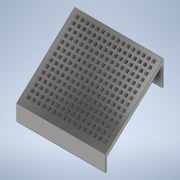
# Autodesk Inventor part: Rejilla_4x4mm
Saved by Autodesk Inventor 2021 (Build 250183000, 183)
## iProperties
Created: 2021-06-27
Part Number: Rejilla_4x4mm
Material: Acero inoxidable
Document SubType Name: Modeling
Designer: artur
Density: 8 g/cm^3
Appearance: Acero - Pulido
Mass: 658.868 g
Surface Area: 625.183 cm^2
Volume: 82.3585 cm^3
Author: artur
Autodesk Inventor part; units mm, degrees
ref_plane "YZ Plane" through (0, 0, 0) normal (1, 0, 0) x (0, 1, 0)
ref_plane "XZ Plane" through (0, 0, 0) normal (0, 1, 0) x (-1, 0, 0)
ref_plane "XY Plane" through (0, 0, 0) normal (0, 0, 1) x (1, 0, 0)
sketch "Boceto6" plane through (-46.053, -27.9809, 0) normal (0, 0, 1) x (1, 0, 0)
  line L0 (118.929, 0) -> (171.1141, 0) construction
  line L1 (-1.0005, -0.9307) -> (-79.0081, -0.9307) construction
  line L2 (-1.0005, -0.9307) -> (89.9995, 83.721)
  line L3 (-1.0005, -0.9307) -> (-1.0005, -25.8991)
  line L4 (-1.0005, -25.8991) -> (0.9995, -25.8991)
  line L5 (0.9995, -25.8991) -> (0.9995, -5.8991)
  line L6 (80.5422, 57.5078) -> (86.2007, 57.5078)
  line L7 (89.9995, 83.721) -> (89.9995, 45.0316)
  line L8 (89.9995, 45.0316) -> (87.9995, 45.0316)
  line L9 (87.9995, 45.0316) -> (87.9995, 75.0316)
  line L10 (0.9995, -5.8991) -> (87.9995, 75.0316)
  dimension "d69" = 137.07
  dimension "d66" = 2
  dimension "d65" = 5
  dimension "d64" = 30
  dimension "d62" = 2
  dimension "d68" = 5
  dimension "d67" = 20
  dimension "d93" = 89
  constraints: 22 end point, 4 horizontal, 2 perpendicular, 2 vertical
  measures "d69" angle of L1 L2
  measures "d66" distance between parallel lines of L5 L3
  measures "d65" distance from line of L2 L9.end
  measures "d64" distance of L8.end L9.end
  measures "d62" distance between parallel lines of L7 L9
  measures "d68" distance from line of L2 L5.end
  measures "d67" distance of L4.end L5.end
  measures "d93" distance between parallel lines of L3 L9
extrude "Extrusión5" add sketch "Boceto6" along normal blind 139
sketch "Boceto7" plane through (-47.0535, -28.9116, 139) normal (-0.6811, 0.7322, 0) x (0.7322, 0.6811, 0)
  line L0 (118.2856, 131) -> (114.2856, 131)
  line L1 (114.2856, 131) -> (114.2856, 127)
  line L2 (114.2856, 127) -> (118.2856, 127)
  line L3 (118.2856, 127) -> (118.2856, 131)
  line L4 (124.2856, 139) -> (124.2856, 0) projected
  line L5 (124.2856, 139) -> (0, 139) projected
  line L6 (118.2856, 123) -> (114.2856, 123)
  line L7 (114.2856, 123) -> (114.2856, 119)
  line L8 (114.2856, 119) -> (118.2856, 119)
  line L9 (118.2856, 119) -> (118.2856, 123)
  line L10 (118.2856, 115) -> (114.2856, 115)
  line L11 (114.2856, 115) -> (114.2856, 111)
  line L12 (114.2856, 111) -> (118.2856, 111)
  line L13 (118.2856, 111) -> (118.2856, 115)
  line L14 (118.2856, 107) -> (114.2856, 107)
  line L15 (114.2856, 107) -> (114.2856, 103)
  line L16 (114.2856, 103) -> (118.2856, 103)
  line L17 (118.2856, 103) -> (118.2856, 107)
  line L18 (118.2856, 99) -> (114.2856, 99)
  line L19 (114.2856, 99) -> (114.2856, 95)
  line L20 (114.2856, 95) -> (118.2856, 95)
  line L21 (118.2856, 95) -> (118.2856, 99)
  line L22 (118.2856, 91) -> (114.2856, 91)
  line L23 (114.2856, 91) -> (114.2856, 87)
  line L24 (114.2856, 87) -> (118.2856, 87)
  line L25 (118.2856, 87) -> (118.2856, 91)
  line L26 (118.2856, 83) -> (114.2856, 83)
  line L27 (114.2856, 83) -> (114.2856, 79)
  line L28 (114.2856, 79) -> (118.2856, 79)
  line L29 (118.2856, 79) -> (118.2856, 83)
  line L30 (118.2856, 75) -> (114.2856, 75)
  line L31 (114.2856, 75) -> (114.2856, 71)
  line L32 (114.2856, 71) -> (118.2856, 71)
  line L33 (118.2856, 71) -> (118.2856, 75)
  line L34 (118.2856, 67) -> (114.2856, 67)
  line L35 (114.2856, 67) -> (114.2856, 63)
  line L36 (114.2856, 63) -> (118.2856, 63)
  line L37 (118.2856, 63) -> (118.2856, 67)
  line L38 (118.2856, 59) -> (114.2856, 59)
  line L39 (114.2856, 59) -> (114.2856, 55)
  line L40 (114.2856, 55) -> (118.2856, 55)
  line L41 (118.2856, 55) -> (118.2856, 59)
  line L42 (118.2856, 51) -> (114.2856, 51)
  line L43 (114.2856, 51) -> (114.2856, 47)
  line L44 (114.2856, 47) -> (118.2856, 47)
  line L45 (118.2856, 47) -> (118.2856, 51)
  line L46 (118.2856, 43) -> (114.2856, 43)
  line L47 (114.2856, 43) -> (114.2856, 39)
  line L48 (114.2856, 39) -> (118.2856, 39)
  line L49 (118.2856, 39) -> (118.2856, 43)
  line L50 (118.2856, 35) -> (114.2856, 35)
  line L51 (114.2856, 35) -> (114.2856, 31)
  line L52 (114.2856, 31) -> (118.2856, 31)
  line L53 (118.2856, 31) -> (118.2856, 35)
  line L54 (118.2856, 27) -> (114.2856, 27)
  line L55 (114.2856, 27) -> (114.2856, 23)
  line L56 (114.2856, 23) -> (118.2856, 23)
  line L57 (118.2856, 23) -> (118.2856, 27)
  line L58 (118.2856, 19) -> (114.2856, 19)
  line L59 (114.2856, 19) -> (114.2856, 15)
  line L60 (114.2856, 15) -> (118.2856, 15)
  line L61 (118.2856, 15) -> (118.2856, 19)
  line L62 (118.2856, 11) -> (114.2856, 11)
  line L63 (114.2856, 11) -> (114.2856, 7)
  line L64 (114.2856, 7) -> (118.2856, 7)
  line L65 (118.2856, 7) -> (118.2856, 11)
  line L66 (110.2856, 127) -> (110.2856, 131)
  line L67 (110.2856, 131) -> (106.2856, 131)
  line L68 (106.2856, 131) -> (106.2856, 127)
  line L69 (106.2856, 123) -> (106.2856, 119)
  line L70 (106.2856, 119) -> (110.2856, 119)
  line L71 (110.2856, 119) -> (110.2856, 123)
  line L72 (110.2856, 115) -> (106.2856, 115)
  line L73 (110.2856, 111) -> (110.2856, 115)
  line L74 (106.2856, 115) -> (106.2856, 111)
  line L75 (106.2856, 111) -> (110.2856, 111)
  line L76 (110.2856, 107) -> (106.2856, 107)
  line L77 (106.2856, 103) -> (110.2856, 103)
  line L78 (106.2856, 107) -> (106.2856, 103)
  line L79 (110.2856, 103) -> (110.2856, 107)
  line L80 (106.2856, 127) -> (110.2856, 127)
  line L81 (110.2856, 123) -> (106.2856, 123)
  line L82 (110.2856, 99) -> (106.2856, 99)
  line L83 (106.2856, 99) -> (106.2856, 95)
  line L84 (110.2856, 95) -> (110.2856, 99)
  line L85 (110.2856, 91) -> (106.2856, 91)
  line L86 (106.2856, 87) -> (110.2856, 87)
  line L87 (110.2856, 87) -> (110.2856, 91)
  line L88 (106.2856, 91) -> (106.2856, 87)
  line L89 (106.2856, 95) -> (110.2856, 95)
  line L90 (110.2856, 83) -> (106.2856, 83)
  line L91 (106.2856, 83) -> (106.2856, 79)
  line L92 (110.2856, 79) -> (110.2856, 83)
  line L93 (106.2856, 79) -> (110.2856, 79)
  line L94 (110.2856, 75) -> (106.2856, 75)
  line L95 (106.2856, 75) -> (106.2856, 71)
  line L96 (110.2856, 71) -> (110.2856, 75)
  line L97 (106.2856, 71) -> (110.2856, 71)
  line L98 (106.2856, 63) -> (110.2856, 63)
  line L99 (110.2856, 63) -> (110.2856, 67)
  line L100 (106.2856, 67) -> (106.2856, 63)
  line L101 (110.2856, 67) -> (106.2856, 67)
  line L102 (110.2856, 59) -> (106.2856, 59)
  line L103 (106.2856, 59) -> (106.2856, 55)
  line L104 (110.2856, 55) -> (110.2856, 59)
  line L105 (106.2856, 55) -> (110.2856, 55)
  line L106 (110.2856, 51) -> (106.2856, 51)
  line L107 (106.2856, 51) -> (106.2856, 47)
  line L108 (106.2856, 47) -> (110.2856, 47)
  line L109 (110.2856, 47) -> (110.2856, 51)
  line L110 (110.2856, 43) -> (106.2856, 43)
  line L111 (106.2856, 43) -> (106.2856, 39)
  line L112 (110.2856, 39) -> (110.2856, 43)
  line L113 (106.2856, 39) -> (110.2856, 39)
  line L114 (110.2856, 35) -> (106.2856, 35)
  line L115 (110.2856, 31) -> (110.2856, 35)
  line L116 (106.2856, 31) -> (110.2856, 31)
  line L117 (106.2856, 35) -> (106.2856, 31)
  line L118 (110.2856, 27) -> (106.2856, 27)
  line L119 (106.2856, 27) -> (106.2856, 23)
  line L120 (110.2856, 23) -> (110.2856, 27)
  line L121 (106.2856, 23) -> (110.2856, 23)
  line L122 (110.2856, 19) -> (106.2856, 19)
  line L123 (106.2856, 19) -> (106.2856, 15)
  line L124 (106.2856, 15) -> (110.2856, 15)
  line L125 (110.2856, 15) -> (110.2856, 19)
  line L126 (110.2856, 11) -> (106.2856, 11)
  line L127 (106.2856, 11) -> (106.2856, 7)
  line L128 (106.2856, 7) -> (110.2856, 7)
  line L129 (110.2856, 7) -> (110.2856, 11)
  line L130 (102.2856, 127) -> (102.2856, 131)
  line L131 (102.2856, 131) -> (98.2856, 131)
  line L132 (98.2856, 131) -> (98.2856, 127)
  line L133 (98.2856, 123) -> (98.2856, 119)
  line L134 (98.2856, 119) -> (102.2856, 119)
  line L135 (102.2856, 119) -> (102.2856, 123)
  line L136 (102.2856, 115) -> (98.2856, 115)
  line L137 (102.2856, 111) -> (102.2856, 115)
  line L138 (98.2856, 115) -> (98.2856, 111)
  line L139 (98.2856, 111) -> (102.2856, 111)
  line L140 (102.2856, 107) -> (98.2856, 107)
  line L141 (98.2856, 103) -> (102.2856, 103)
  line L142 (98.2856, 107) -> (98.2856, 103)
  line L143 (102.2856, 103) -> (102.2856, 107)
  line L144 (98.2856, 127) -> (102.2856, 127)
  line L145 (102.2856, 123) -> (98.2856, 123)
  line L146 (102.2856, 99) -> (98.2856, 99)
  line L147 (98.2856, 99) -> (98.2856, 95)
  line L148 (102.2856, 95) -> (102.2856, 99)
  line L149 (102.2856, 91) -> (98.2856, 91)
  line L150 (98.2856, 87) -> (102.2856, 87)
  line L151 (102.2856, 87) -> (102.2856, 91)
  line L152 (98.2856, 91) -> (98.2856, 87)
  line L153 (98.2856, 95) -> (102.2856, 95)
  line L154 (102.2856, 83) -> (98.2856, 83)
  line L155 (98.2856, 83) -> (98.2856, 79)
  line L156 (102.2856, 79) -> (102.2856, 83)
  line L157 (98.2856, 79) -> (102.2856, 79)
  line L158 (102.2856, 75) -> (98.2856, 75)
  line L159 (98.2856, 75) -> (98.2856, 71)
  line L160 (102.2856, 71) -> (102.2856, 75)
  line L161 (98.2856, 71) -> (102.2856, 71)
  line L162 (98.2856, 63) -> (102.2856, 63)
  line L163 (102.2856, 63) -> (102.2856, 67)
  line L164 (98.2856, 67) -> (98.2856, 63)
  line L165 (102.2856, 67) -> (98.2856, 67)
  line L166 (102.2856, 59) -> (98.2856, 59)
  line L167 (98.2856, 59) -> (98.2856, 55)
  line L168 (102.2856, 55) -> (102.2856, 59)
  line L169 (98.2856, 55) -> (102.2856, 55)
  line L170 (102.2856, 51) -> (98.2856, 51)
  line L171 (98.2856, 51) -> (98.2856, 47)
  line L172 (98.2856, 47) -> (102.2856, 47)
  line L173 (102.2856, 47) -> (102.2856, 51)
  line L174 (102.2856, 43) -> (98.2856, 43)
  line L175 (98.2856, 43) -> (98.2856, 39)
  line L176 (102.2856, 39) -> (102.2856, 43)
  line L177 (98.2856, 39) -> (102.2856, 39)
  line L178 (102.2856, 35) -> (98.2856, 35)
  line L179 (102.2856, 31) -> (102.2856, 35)
  line L180 (98.2856, 31) -> (102.2856, 31)
  line L181 (98.2856, 35) -> (98.2856, 31)
  line L182 (102.2856, 27) -> (98.2856, 27)
  line L183 (98.2856, 27) -> (98.2856, 23)
  line L184 (102.2856, 23) -> (102.2856, 27)
  line L185 (98.2856, 23) -> (102.2856, 23)
  line L186 (102.2856, 19) -> (98.2856, 19)
  line L187 (98.2856, 19) -> (98.2856, 15)
  line L188 (98.2856, 15) -> (102.2856, 15)
  line L189 (102.2856, 15) -> (102.2856, 19)
  line L190 (102.2856, 11) -> (98.2856, 11)
  line L191 (98.2856, 11) -> (98.2856, 7)
  line L192 (98.2856, 7) -> (102.2856, 7)
  line L193 (102.2856, 7) -> (102.2856, 11)
  line L194 (94.2856, 127) -> (94.2856, 131)
  line L195 (94.2856, 131) -> (90.2856, 131)
  line L196 (90.2856, 131) -> (90.2856, 127)
  line L197 (90.2856, 123) -> (90.2856, 119)
  line L198 (90.2856, 119) -> (94.2856, 119)
  line L199 (94.2856, 119) -> (94.2856, 123)
  line L200 (94.2856, 115) -> (90.2856, 115)
  line L201 (94.2856, 111) -> (94.2856, 115)
  line L202 (90.2856, 115) -> (90.2856, 111)
  line L203 (90.2856, 111) -> (94.2856, 111)
  line L204 (94.2856, 107) -> (90.2856, 107)
  line L205 (90.2856, 103) -> (94.2856, 103)
  line L206 (90.2856, 107) -> (90.2856, 103)
  line L207 (94.2856, 103) -> (94.2856, 107)
  line L208 (90.2856, 127) -> (94.2856, 127)
  line L209 (94.2856, 123) -> (90.2856, 123)
  line L210 (94.2856, 99) -> (90.2856, 99)
  line L211 (90.2856, 99) -> (90.2856, 95)
  line L212 (94.2856, 95) -> (94.2856, 99)
  line L213 (94.2856, 91) -> (90.2856, 91)
  line L214 (90.2856, 87) -> (94.2856, 87)
  line L215 (94.2856, 87) -> (94.2856, 91)
  line L216 (90.2856, 91) -> (90.2856, 87)
  line L217 (90.2856, 95) -> (94.2856, 95)
  line L218 (94.2856, 83) -> (90.2856, 83)
  line L219 (90.2856, 83) -> (90.2856, 79)
  line L220 (94.2856, 79) -> (94.2856, 83)
  line L221 (90.2856, 79) -> (94.2856, 79)
  line L222 (94.2856, 75) -> (90.2856, 75)
  line L223 (90.2856, 75) -> (90.2856, 71)
  line L224 (94.2856, 71) -> (94.2856, 75)
  line L225 (90.2856, 71) -> (94.2856, 71)
  line L226 (90.2856, 63) -> (94.2856, 63)
  line L227 (94.2856, 63) -> (94.2856, 67)
  line L228 (90.2856, 67) -> (90.2856, 63)
  line L229 (94.2856, 67) -> (90.2856, 67)
  line L230 (94.2856, 59) -> (90.2856, 59)
  line L231 (90.2856, 59) -> (90.2856, 55)
  line L232 (94.2856, 55) -> (94.2856, 59)
  line L233 (90.2856, 55) -> (94.2856, 55)
  line L234 (94.2856, 51) -> (90.2856, 51)
  line L235 (90.2856, 51) -> (90.2856, 47)
  line L236 (90.2856, 47) -> (94.2856, 47)
  line L237 (94.2856, 47) -> (94.2856, 51)
  line L238 (94.2856, 43) -> (90.2856, 43)
  line L239 (90.2856, 43) -> (90.2856, 39)
  line L240 (94.2856, 39) -> (94.2856, 43)
  line L241 (90.2856, 39) -> (94.2856, 39)
  line L242 (94.2856, 35) -> (90.2856, 35)
  line L243 (94.2856, 31) -> (94.2856, 35)
  line L244 (90.2856, 31) -> (94.2856, 31)
  line L245 (90.2856, 35) -> (90.2856, 31)
  line L246 (94.2856, 27) -> (90.2856, 27)
  line L247 (90.2856, 27) -> (90.2856, 23)
  line L248 (94.2856, 23) -> (94.2856, 27)
  line L249 (90.2856, 23) -> (94.2856, 23)
  line L250 (94.2856, 19) -> (90.2856, 19)
  line L251 (90.2856, 19) -> (90.2856, 15)
  line L252 (90.2856, 15) -> (94.2856, 15)
  line L253 (94.2856, 15) -> (94.2856, 19)
  line L254 (94.2856, 11) -> (90.2856, 11)
  line L255 (90.2856, 11) -> (90.2856, 7)
  line L256 (90.2856, 7) -> (94.2856, 7)
  line L257 (94.2856, 7) -> (94.2856, 11)
  line L258 (86.2856, 127) -> (86.2856, 131)
  line L259 (86.2856, 131) -> (82.2856, 131)
  line L260 (82.2856, 131) -> (82.2856, 127)
  line L261 (82.2856, 123) -> (82.2856, 119)
  line L262 (82.2856, 119) -> (86.2856, 119)
  line L263 (86.2856, 119) -> (86.2856, 123)
  line L264 (86.2856, 115) -> (82.2856, 115)
  line L265 (86.2856, 111) -> (86.2856, 115)
  line L266 (82.2856, 115) -> (82.2856, 111)
  line L267 (82.2856, 111) -> (86.2856, 111)
  line L268 (86.2856, 107) -> (82.2856, 107)
  line L269 (82.2856, 103) -> (86.2856, 103)
  line L270 (82.2856, 107) -> (82.2856, 103)
  line L271 (86.2856, 103) -> (86.2856, 107)
  line L272 (82.2856, 127) -> (86.2856, 127)
  line L273 (86.2856, 123) -> (82.2856, 123)
  line L274 (86.2856, 99) -> (82.2856, 99)
  line L275 (82.2856, 99) -> (82.2856, 95)
  line L276 (86.2856, 95) -> (86.2856, 99)
  line L277 (86.2856, 91) -> (82.2856, 91)
  line L278 (82.2856, 87) -> (86.2856, 87)
  line L279 (86.2856, 87) -> (86.2856, 91)
  line L280 (82.2856, 91) -> (82.2856, 87)
  line L281 (82.2856, 95) -> (86.2856, 95)
  line L282 (86.2856, 83) -> (82.2856, 83)
  line L283 (82.2856, 83) -> (82.2856, 79)
  line L284 (86.2856, 79) -> (86.2856, 83)
  line L285 (82.2856, 79) -> (86.2856, 79)
  line L286 (86.2856, 75) -> (82.2856, 75)
  line L287 (82.2856, 75) -> (82.2856, 71)
  line L288 (86.2856, 71) -> (86.2856, 75)
  line L289 (82.2856, 71) -> (86.2856, 71)
  line L290 (82.2856, 63) -> (86.2856, 63)
  line L291 (86.2856, 63) -> (86.2856, 67)
  line L292 (82.2856, 67) -> (82.2856, 63)
  line L293 (86.2856, 67) -> (82.2856, 67)
  line L294 (86.2856, 59) -> (82.2856, 59)
  line L295 (82.2856, 59) -> (82.2856, 55)
  line L296 (86.2856, 55) -> (86.2856, 59)
  line L297 (82.2856, 55) -> (86.2856, 55)
  line L298 (86.2856, 51) -> (82.2856, 51)
  line L299 (82.2856, 51) -> (82.2856, 47)
  line L300 (82.2856, 47) -> (86.2856, 47)
  line L301 (86.2856, 47) -> (86.2856, 51)
  line L302 (86.2856, 43) -> (82.2856, 43)
  line L303 (82.2856, 43) -> (82.2856, 39)
  line L304 (86.2856, 39) -> (86.2856, 43)
  line L305 (82.2856, 39) -> (86.2856, 39)
  line L306 (86.2856, 35) -> (82.2856, 35)
  line L307 (86.2856, 31) -> (86.2856, 35)
  line L308 (82.2856, 31) -> (86.2856, 31)
  line L309 (82.2856, 35) -> (82.2856, 31)
  line L310 (86.2856, 27) -> (82.2856, 27)
  line L311 (82.2856, 27) -> (82.2856, 23)
  line L312 (86.2856, 23) -> (86.2856, 27)
  line L313 (82.2856, 23) -> (86.2856, 23)
  line L314 (86.2856, 19) -> (82.2856, 19)
  line L315 (82.2856, 19) -> (82.2856, 15)
  line L316 (82.2856, 15) -> (86.2856, 15)
  line L317 (86.2856, 15) -> (86.2856, 19)
  line L318 (86.2856, 11) -> (82.2856, 11)
  line L319 (82.2856, 11) -> (82.2856, 7)
  line L320 (82.2856, 7) -> (86.2856, 7)
  line L321 (86.2856, 7) -> (86.2856, 11)
  line L322 (78.2856, 127) -> (78.2856, 131)
  line L323 (78.2856, 131) -> (74.2856, 131)
  line L324 (74.2856, 131) -> (74.2856, 127)
  line L325 (74.2856, 123) -> (74.2856, 119)
  line L326 (74.2856, 119) -> (78.2856, 119)
  line L327 (78.2856, 119) -> (78.2856, 123)
  line L328 (78.2856, 115) -> (74.2856, 115)
  line L329 (78.2856, 111) -> (78.2856, 115)
  line L330 (74.2856, 115) -> (74.2856, 111)
  line L331 (74.2856, 111) -> (78.2856, 111)
  line L332 (78.2856, 107) -> (74.2856, 107)
  line L333 (74.2856, 103) -> (78.2856, 103)
  line L334 (74.2856, 107) -> (74.2856, 103)
  line L335 (78.2856, 103) -> (78.2856, 107)
  line L336 (74.2856, 127) -> (78.2856, 127)
  line L337 (78.2856, 123) -> (74.2856, 123)
  line L338 (78.2856, 99) -> (74.2856, 99)
  line L339 (74.2856, 99) -> (74.2856, 95)
  line L340 (78.2856, 95) -> (78.2856, 99)
  line L341 (78.2856, 91) -> (74.2856, 91)
  line L342 (74.2856, 87) -> (78.2856, 87)
  line L343 (78.2856, 87) -> (78.2856, 91)
  line L344 (74.2856, 91) -> (74.2856, 87)
  line L345 (74.2856, 95) -> (78.2856, 95)
  line L346 (78.2856, 83) -> (74.2856, 83)
  line L347 (74.2856, 83) -> (74.2856, 79)
  line L348 (78.2856, 79) -> (78.2856, 83)
  line L349 (74.2856, 79) -> (78.2856, 79)
  line L350 (78.2856, 75) -> (74.2856, 75)
  line L351 (74.2856, 75) -> (74.2856, 71)
  line L352 (78.2856, 71) -> (78.2856, 75)
  line L353 (74.2856, 71) -> (78.2856, 71)
  line L354 (74.2856, 63) -> (78.2856, 63)
  line L355 (78.2856, 63) -> (78.2856, 67)
  line L356 (74.2856, 67) -> (74.2856, 63)
  line L357 (78.2856, 67) -> (74.2856, 67)
  line L358 (78.2856, 59) -> (74.2856, 59)
  line L359 (74.2856, 59) -> (74.2856, 55)
  line L360 (78.2856, 55) -> (78.2856, 59)
  line L361 (74.2856, 55) -> (78.2856, 55)
  line L362 (78.2856, 51) -> (74.2856, 51)
  line L363 (74.2856, 51) -> (74.2856, 47)
  line L364 (74.2856, 47) -> (78.2856, 47)
  line L365 (78.2856, 47) -> (78.2856, 51)
  line L366 (78.2856, 43) -> (74.2856, 43)
  line L367 (74.2856, 43) -> (74.2856, 39)
  line L368 (78.2856, 39) -> (78.2856, 43)
  line L369 (74.2856, 39) -> (78.2856, 39)
  line L370 (78.2856, 35) -> (74.2856, 35)
  line L371 (78.2856, 31) -> (78.2856, 35)
  line L372 (74.2856, 31) -> (78.2856, 31)
  line L373 (74.2856, 35) -> (74.2856, 31)
  line L374 (78.2856, 27) -> (74.2856, 27)
  line L375 (74.2856, 27) -> (74.2856, 23)
  line L376 (78.2856, 23) -> (78.2856, 27)
  line L377 (74.2856, 23) -> (78.2856, 23)
  line L378 (78.2856, 19) -> (74.2856, 19)
  line L379 (74.2856, 19) -> (74.2856, 15)
  line L380 (74.2856, 15) -> (78.2856, 15)
  line L381 (78.2856, 15) -> (78.2856, 19)
  line L382 (78.2856, 11) -> (74.2856, 11)
  line L383 (74.2856, 11) -> (74.2856, 7)
  line L384 (74.2856, 7) -> (78.2856, 7)
  line L385 (78.2856, 7) -> (78.2856, 11)
  line L386 (70.2856, 127) -> (70.2856, 131)
  line L387 (70.2856, 131) -> (66.2856, 131)
  line L388 (66.2856, 131) -> (66.2856, 127)
  line L389 (66.2856, 123) -> (66.2856, 119)
  line L390 (66.2856, 119) -> (70.2856, 119)
  line L391 (70.2856, 119) -> (70.2856, 123)
  line L392 (70.2856, 115) -> (66.2856, 115)
  line L393 (70.2856, 111) -> (70.2856, 115)
  line L394 (66.2856, 115) -> (66.2856, 111)
  line L395 (66.2856, 111) -> (70.2856, 111)
  line L396 (70.2856, 107) -> (66.2856, 107)
  line L397 (66.2856, 103) -> (70.2856, 103)
  line L398 (66.2856, 107) -> (66.2856, 103)
  line L399 (70.2856, 103) -> (70.2856, 107)
  line L400 (66.2856, 127) -> (70.2856, 127)
  line L401 (70.2856, 123) -> (66.2856, 123)
  line L402 (70.2856, 99) -> (66.2856, 99)
  line L403 (66.2856, 99) -> (66.2856, 95)
  line L404 (70.2856, 95) -> (70.2856, 99)
  line L405 (70.2856, 91) -> (66.2856, 91)
  line L406 (66.2856, 87) -> (70.2856, 87)
  line L407 (70.2856, 87) -> (70.2856, 91)
  line L408 (66.2856, 91) -> (66.2856, 87)
  line L409 (66.2856, 95) -> (70.2856, 95)
  line L410 (70.2856, 83) -> (66.2856, 83)
  line L411 (66.2856, 83) -> (66.2856, 79)
  line L412 (70.2856, 79) -> (70.2856, 83)
  line L413 (66.2856, 79) -> (70.2856, 79)
  line L414 (70.2856, 75) -> (66.2856, 75)
  line L415 (66.2856, 75) -> (66.2856, 71)
  line L416 (70.2856, 71) -> (70.2856, 75)
  line L417 (66.2856, 71) -> (70.2856, 71)
  line L418 (66.2856, 63) -> (70.2856, 63)
  line L419 (70.2856, 63) -> (70.2856, 67)
  line L420 (66.2856, 67) -> (66.2856, 63)
  line L421 (70.2856, 67) -> (66.2856, 67)
  line L422 (70.2856, 59) -> (66.2856, 59)
  line L423 (66.2856, 59) -> (66.2856, 55)
  line L424 (70.2856, 55) -> (70.2856, 59)
  line L425 (66.2856, 55) -> (70.2856, 55)
  line L426 (70.2856, 51) -> (66.2856, 51)
  line L427 (66.2856, 51) -> (66.2856, 47)
  line L428 (66.2856, 47) -> (70.2856, 47)
  line L429 (70.2856, 47) -> (70.2856, 51)
  line L430 (70.2856, 43) -> (66.2856, 43)
  line L431 (66.2856, 43) -> (66.2856, 39)
  line L432 (70.2856, 39) -> (70.2856, 43)
  line L433 (66.2856, 39) -> (70.2856, 39)
  line L434 (70.2856, 35) -> (66.2856, 35)
  line L435 (70.2856, 31) -> (70.2856, 35)
  line L436 (66.2856, 31) -> (70.2856, 31)
  line L437 (66.2856, 35) -> (66.2856, 31)
  line L438 (70.2856, 27) -> (66.2856, 27)
  line L439 (66.2856, 27) -> (66.2856, 23)
  line L440 (70.2856, 23) -> (70.2856, 27)
  line L441 (66.2856, 23) -> (70.2856, 23)
  line L442 (70.2856, 19) -> (66.2856, 19)
  line L443 (66.2856, 19) -> (66.2856, 15)
  line L444 (66.2856, 15) -> (70.2856, 15)
  line L445 (70.2856, 15) -> (70.2856, 19)
  line L446 (70.2856, 11) -> (66.2856, 11)
  line L447 (66.2856, 11) -> (66.2856, 7)
  line L448 (66.2856, 7) -> (70.2856, 7)
  line L449 (70.2856, 7) -> (70.2856, 11)
  line L450 (62.2856, 127) -> (62.2856, 131)
  line L451 (62.2856, 131) -> (58.2856, 131)
  line L452 (58.2856, 131) -> (58.2856, 127)
  line L453 (58.2856, 123) -> (58.2856, 119)
  line L454 (58.2856, 119) -> (62.2856, 119)
  line L455 (62.2856, 119) -> (62.2856, 123)
  line L456 (62.2856, 115) -> (58.2856, 115)
  line L457 (62.2856, 111) -> (62.2856, 115)
  line L458 (58.2856, 115) -> (58.2856, 111)
  line L459 (58.2856, 111) -> (62.2856, 111)
  line L460 (62.2856, 107) -> (58.2856, 107)
  line L461 (58.2856, 103) -> (62.2856, 103)
  line L462 (58.2856, 107) -> (58.2856, 103)
  line L463 (62.2856, 103) -> (62.2856, 107)
  line L464 (58.2856, 127) -> (62.2856, 127)
  line L465 (62.2856, 123) -> (58.2856, 123)
  line L466 (62.2856, 99) -> (58.2856, 99)
  line L467 (58.2856, 99) -> (58.2856, 95)
  line L468 (62.2856, 95) -> (62.2856, 99)
  line L469 (62.2856, 91) -> (58.2856, 91)
  line L470 (58.2856, 87) -> (62.2856, 87)
  line L471 (62.2856, 87) -> (62.2856, 91)
  line L472 (58.2856, 91) -> (58.2856, 87)
  line L473 (58.2856, 95) -> (62.2856, 95)
  line L474 (62.2856, 83) -> (58.2856, 83)
  line L475 (58.2856, 83) -> (58.2856, 79)
  line L476 (62.2856, 79) -> (62.2856, 83)
  line L477 (58.2856, 79) -> (62.2856, 79)
  line L478 (62.2856, 75) -> (58.2856, 75)
  line L479 (58.2856, 75) -> (58.2856, 71)
  line L480 (62.2856, 71) -> (62.2856, 75)
  line L481 (58.2856, 71) -> (62.2856, 71)
  line L482 (58.2856, 63) -> (62.2856, 63)
  line L483 (62.2856, 63) -> (62.2856, 67)
  line L484 (58.2856, 67) -> (58.2856, 63)
  line L485 (62.2856, 67) -> (58.2856, 67)
  line L486 (62.2856, 59) -> (58.2856, 59)
  line L487 (58.2856, 59) -> (58.2856, 55)
  line L488 (62.2856, 55) -> (62.2856, 59)
  line L489 (58.2856, 55) -> (62.2856, 55)
  line L490 (62.2856, 51) -> (58.2856, 51)
  line L491 (58.2856, 51) -> (58.2856, 47)
  line L492 (58.2856, 47) -> (62.2856, 47)
  line L493 (62.2856, 47) -> (62.2856, 51)
  line L494 (62.2856, 43) -> (58.2856, 43)
  line L495 (58.2856, 43) -> (58.2856, 39)
  line L496 (62.2856, 39) -> (62.2856, 43)
  line L497 (58.2856, 39) -> (62.2856, 39)
  line L498 (62.2856, 35) -> (58.2856, 35)
  line L499 (62.2856, 31) -> (62.2856, 35)
  line L500 (58.2856, 31) -> (62.2856, 31)
  line L501 (58.2856, 35) -> (58.2856, 31)
  line L502 (62.2856, 27) -> (58.2856, 27)
  line L503 (58.2856, 27) -> (58.2856, 23)
  line L504 (62.2856, 23) -> (62.2856, 27)
  line L505 (58.2856, 23) -> (62.2856, 23)
  line L506 (62.2856, 19) -> (58.2856, 19)
  line L507 (58.2856, 19) -> (58.2856, 15)
  line L508 (58.2856, 15) -> (62.2856, 15)
  line L509 (62.2856, 15) -> (62.2856, 19)
  line L510 (62.2856, 11) -> (58.2856, 11)
  line L511 (58.2856, 11) -> (58.2856, 7)
  line L512 (58.2856, 7) -> (62.2856, 7)
  line L513 (62.2856, 7) -> (62.2856, 11)
  line L514 (54.2856, 127) -> (54.2856, 131)
  line L515 (54.2856, 131) -> (50.2856, 131)
  line L516 (50.2856, 131) -> (50.2856, 127)
  line L517 (50.2856, 123) -> (50.2856, 119)
  line L518 (50.2856, 119) -> (54.2856, 119)
  line L519 (54.2856, 119) -> (54.2856, 123)
  line L520 (54.2856, 115) -> (50.2856, 115)
  line L521 (54.2856, 111) -> (54.2856, 115)
  line L522 (50.2856, 115) -> (50.2856, 111)
  line L523 (50.2856, 111) -> (54.2856, 111)
  line L524 (54.2856, 107) -> (50.2856, 107)
  line L525 (50.2856, 103) -> (54.2856, 103)
  line L526 (50.2856, 107) -> (50.2856, 103)
  line L527 (54.2856, 103) -> (54.2856, 107)
  line L528 (50.2856, 127) -> (54.2856, 127)
  line L529 (54.2856, 123) -> (50.2856, 123)
  line L530 (54.2856, 99) -> (50.2856, 99)
  line L531 (50.2856, 99) -> (50.2856, 95)
  line L532 (54.2856, 95) -> (54.2856, 99)
  line L533 (54.2856, 91) -> (50.2856, 91)
  line L534 (50.2856, 87) -> (54.2856, 87)
  line L535 (54.2856, 87) -> (54.2856, 91)
  line L536 (50.2856, 91) -> (50.2856, 87)
  line L537 (50.2856, 95) -> (54.2856, 95)
  line L538 (54.2856, 83) -> (50.2856, 83)
  line L539 (50.2856, 83) -> (50.2856, 79)
  line L540 (54.2856, 79) -> (54.2856, 83)
  line L541 (50.2856, 79) -> (54.2856, 79)
  line L542 (54.2856, 75) -> (50.2856, 75)
  line L543 (50.2856, 75) -> (50.2856, 71)
  line L544 (54.2856, 71) -> (54.2856, 75)
  line L545 (50.2856, 71) -> (54.2856, 71)
  line L546 (50.2856, 63) -> (54.2856, 63)
  line L547 (54.2856, 63) -> (54.2856, 67)
  line L548 (50.2856, 67) -> (50.2856, 63)
  line L549 (54.2856, 67) -> (50.2856, 67)
  line L550 (54.2856, 59) -> (50.2856, 59)
  line L551 (50.2856, 59) -> (50.2856, 55)
  line L552 (54.2856, 55) -> (54.2856, 59)
  line L553 (50.2856, 55) -> (54.2856, 55)
  line L554 (54.2856, 51) -> (50.2856, 51)
  line L555 (50.2856, 51) -> (50.2856, 47)
  line L556 (50.2856, 47) -> (54.2856, 47)
  line L557 (54.2856, 47) -> (54.2856, 51)
  line L558 (54.2856, 43) -> (50.2856, 43)
  line L559 (50.2856, 43) -> (50.2856, 39)
  line L560 (54.2856, 39) -> (54.2856, 43)
  line L561 (50.2856, 39) -> (54.2856, 39)
  line L562 (54.2856, 35) -> (50.2856, 35)
  line L563 (54.2856, 31) -> (54.2856, 35)
  line L564 (50.2856, 31) -> (54.2856, 31)
  line L565 (50.2856, 35) -> (50.2856, 31)
  line L566 (54.2856, 27) -> (50.2856, 27)
  line L567 (50.2856, 27) -> (50.2856, 23)
  line L568 (54.2856, 23) -> (54.2856, 27)
  line L569 (50.2856, 23) -> (54.2856, 23)
  line L570 (54.2856, 19) -> (50.2856, 19)
  line L571 (50.2856, 19) -> (50.2856, 15)
  line L572 (50.2856, 15) -> (54.2856, 15)
  line L573 (54.2856, 15) -> (54.2856, 19)
  line L574 (54.2856, 11) -> (50.2856, 11)
  line L575 (50.2856, 11) -> (50.2856, 7)
  line L576 (50.2856, 7) -> (54.2856, 7)
  line L577 (54.2856, 7) -> (54.2856, 11)
  line L578 (46.2856, 127) -> (46.2856, 131)
  line L579 (46.2856, 131) -> (42.2856, 131)
  line L580 (42.2856, 131) -> (42.2856, 127)
  line L581 (42.2856, 123) -> (42.2856, 119)
  line L582 (42.2856, 119) -> (46.2856, 119)
  line L583 (46.2856, 119) -> (46.2856, 123)
  line L584 (46.2856, 115) -> (42.2856, 115)
  line L585 (46.2856, 111) -> (46.2856, 115)
  line L586 (42.2856, 115) -> (42.2856, 111)
  line L587 (42.2856, 111) -> (46.2856, 111)
  line L588 (46.2856, 107) -> (42.2856, 107)
  line L589 (42.2856, 103) -> (46.2856, 103)
  line L590 (42.2856, 107) -> (42.2856, 103)
  line L591 (46.2856, 103) -> (46.2856, 107)
  line L592 (42.2856, 127) -> (46.2856, 127)
  line L593 (46.2856, 123) -> (42.2856, 123)
  line L594 (46.2856, 99) -> (42.2856, 99)
  line L595 (42.2856, 99) -> (42.2856, 95)
  line L596 (46.2856, 95) -> (46.2856, 99)
  line L597 (46.2856, 91) -> (42.2856, 91)
  line L598 (42.2856, 87) -> (46.2856, 87)
  line L599 (46.2856, 87) -> (46.2856, 91)
  line L600 (42.2856, 91) -> (42.2856, 87)
  line L601 (42.2856, 95) -> (46.2856, 95)
  line L602 (46.2856, 83) -> (42.2856, 83)
  line L603 (42.2856, 83) -> (42.2856, 79)
  line L604 (46.2856, 79) -> (46.2856, 83)
  line L605 (42.2856, 79) -> (46.2856, 79)
  line L606 (46.2856, 75) -> (42.2856, 75)
  line L607 (42.2856, 75) -> (42.2856, 71)
  line L608 (46.2856, 71) -> (46.2856, 75)
  line L609 (42.2856, 71) -> (46.2856, 71)
  line L610 (42.2856, 63) -> (46.2856, 63)
  line L611 (46.2856, 63) -> (46.2856, 67)
  line L612 (42.2856, 67) -> (42.2856, 63)
  line L613 (46.2856, 67) -> (42.2856, 67)
  line L614 (46.2856, 59) -> (42.2856, 59)
  line L615 (42.2856, 59) -> (42.2856, 55)
  line L616 (46.2856, 55) -> (46.2856, 59)
  line L617 (42.2856, 55) -> (46.2856, 55)
  line L618 (46.2856, 51) -> (42.2856, 51)
  line L619 (42.2856, 51) -> (42.2856, 47)
  line L620 (42.2856, 47) -> (46.2856, 47)
  line L621 (46.2856, 47) -> (46.2856, 51)
  line L622 (46.2856, 43) -> (42.2856, 43)
  line L623 (42.2856, 43) -> (42.2856, 39)
  line L624 (46.2856, 39) -> (46.2856, 43)
  line L625 (42.2856, 39) -> (46.2856, 39)
  line L626 (46.2856, 35) -> (42.2856, 35)
  line L627 (46.2856, 31) -> (46.2856, 35)
  line L628 (42.2856, 31) -> (46.2856, 31)
  line L629 (42.2856, 35) -> (42.2856, 31)
  line L630 (46.2856, 27) -> (42.2856, 27)
  line L631 (42.2856, 27) -> (42.2856, 23)
  line L632 (46.2856, 23) -> (46.2856, 27)
  line L633 (42.2856, 23) -> (46.2856, 23)
  line L634 (46.2856, 19) -> (42.2856, 19)
  line L635 (42.2856, 19) -> (42.2856, 15)
  line L636 (42.2856, 15) -> (46.2856, 15)
  line L637 (46.2856, 15) -> (46.2856, 19)
  line L638 (46.2856, 11) -> (42.2856, 11)
  line L639 (42.2856, 11) -> (42.2856, 7)
  line L640 (42.2856, 7) -> (46.2856, 7)
  line L641 (46.2856, 7) -> (46.2856, 11)
  line L642 (38.2856, 127) -> (38.2856, 131)
  line L643 (38.2856, 131) -> (34.2856, 131)
  line L644 (34.2856, 131) -> (34.2856, 127)
  line L645 (34.2856, 123) -> (34.2856, 119)
  line L646 (34.2856, 119) -> (38.2856, 119)
  line L647 (38.2856, 119) -> (38.2856, 123)
  line L648 (38.2856, 115) -> (34.2856, 115)
  line L649 (38.2856, 111) -> (38.2856, 115)
  line L650 (34.2856, 115) -> (34.2856, 111)
  line L651 (34.2856, 111) -> (38.2856, 111)
  line L652 (38.2856, 107) -> (34.2856, 107)
  line L653 (34.2856, 103) -> (38.2856, 103)
  line L654 (34.2856, 107) -> (34.2856, 103)
  line L655 (38.2856, 103) -> (38.2856, 107)
  line L656 (34.2856, 127) -> (38.2856, 127)
  line L657 (38.2856, 123) -> (34.2856, 123)
  line L658 (38.2856, 99) -> (34.2856, 99)
  line L659 (34.2856, 99) -> (34.2856, 95)
  line L660 (38.2856, 95) -> (38.2856, 99)
  line L661 (38.2856, 91) -> (34.2856, 91)
  line L662 (34.2856, 87) -> (38.2856, 87)
  line L663 (38.2856, 87) -> (38.2856, 91)
  line L664 (34.2856, 91) -> (34.2856, 87)
  line L665 (34.2856, 95) -> (38.2856, 95)
  line L666 (38.2856, 83) -> (34.2856, 83)
  line L667 (34.2856, 83) -> (34.2856, 79)
  line L668 (38.2856, 79) -> (38.2856, 83)
  line L669 (34.2856, 79) -> (38.2856, 79)
  line L670 (38.2856, 75) -> (34.2856, 75)
  line L671 (34.2856, 75) -> (34.2856, 71)
  line L672 (38.2856, 71) -> (38.2856, 75)
  line L673 (34.2856, 71) -> (38.2856, 71)
  line L674 (34.2856, 63) -> (38.2856, 63)
  line L675 (38.2856, 63) -> (38.2856, 67)
  line L676 (34.2856, 67) -> (34.2856, 63)
  line L677 (38.2856, 67) -> (34.2856, 67)
  line L678 (38.2856, 59) -> (34.2856, 59)
  line L679 (34.2856, 59) -> (34.2856, 55)
  line L680 (38.2856, 55) -> (38.2856, 59)
  line L681 (34.2856, 55) -> (38.2856, 55)
  line L682 (38.2856, 51) -> (34.2856, 51)
  line L683 (34.2856, 51) -> (34.2856, 47)
  line L684 (34.2856, 47) -> (38.2856, 47)
  line L685 (38.2856, 47) -> (38.2856, 51)
  line L686 (38.2856, 43) -> (34.2856, 43)
  line L687 (34.2856, 43) -> (34.2856, 39)
  line L688 (38.2856, 39) -> (38.2856, 43)
  line L689 (34.2856, 39) -> (38.2856, 39)
  line L690 (38.2856, 35) -> (34.2856, 35)
  line L691 (38.2856, 31) -> (38.2856, 35)
  line L692 (34.2856, 31) -> (38.2856, 31)
  line L693 (34.2856, 35) -> (34.2856, 31)
  line L694 (38.2856, 27) -> (34.2856, 27)
  line L695 (34.2856, 27) -> (34.2856, 23)
  line L696 (38.2856, 23) -> (38.2856, 27)
  line L697 (34.2856, 23) -> (38.2856, 23)
  line L698 (38.2856, 19) -> (34.2856, 19)
  line L699 (34.2856, 19) -> (34.2856, 15)
  line L700 (34.2856, 15) -> (38.2856, 15)
  line L701 (38.2856, 15) -> (38.2856, 19)
  line L702 (38.2856, 11) -> (34.2856, 11)
  line L703 (34.2856, 11) -> (34.2856, 7)
  line L704 (34.2856, 7) -> (38.2856, 7)
  line L705 (38.2856, 7) -> (38.2856, 11)
  line L706 (30.2856, 127) -> (30.2856, 131)
  line L707 (30.2856, 131) -> (26.2856, 131)
  line L708 (26.2856, 131) -> (26.2856, 127)
  line L709 (26.2856, 123) -> (26.2856, 119)
  line L710 (26.2856, 119) -> (30.2856, 119)
  line L711 (30.2856, 119) -> (30.2856, 123)
  line L712 (30.2856, 115) -> (26.2856, 115)
  line L713 (30.2856, 111) -> (30.2856, 115)
  line L714 (26.2856, 115) -> (26.2856, 111)
  line L715 (26.2856, 111) -> (30.2856, 111)
  line L716 (30.2856, 107) -> (26.2856, 107)
  line L717 (26.2856, 103) -> (30.2856, 103)
  line L718 (26.2856, 107) -> (26.2856, 103)
  line L719 (30.2856, 103) -> (30.2856, 107)
  line L720 (26.2856, 127) -> (30.2856, 127)
  line L721 (30.2856, 123) -> (26.2856, 123)
  line L722 (30.2856, 99) -> (26.2856, 99)
  line L723 (26.2856, 99) -> (26.2856, 95)
  line L724 (30.2856, 95) -> (30.2856, 99)
  line L725 (30.2856, 91) -> (26.2856, 91)
  line L726 (26.2856, 87) -> (30.2856, 87)
  line L727 (30.2856, 87) -> (30.2856, 91)
  line L728 (26.2856, 91) -> (26.2856, 87)
  line L729 (26.2856, 95) -> (30.2856, 95)
  line L730 (30.2856, 83) -> (26.2856, 83)
  line L731 (26.2856, 83) -> (26.2856, 79)
  line L732 (30.2856, 79) -> (30.2856, 83)
  line L733 (26.2856, 79) -> (30.2856, 79)
  line L734 (30.2856, 75) -> (26.2856, 75)
  line L735 (26.2856, 75) -> (26.2856, 71)
  line L736 (30.2856, 71) -> (30.2856, 75)
  line L737 (26.2856, 71) -> (30.2856, 71)
  line L738 (26.2856, 63) -> (30.2856, 63)
  line L739 (30.2856, 63) -> (30.2856, 67)
  line L740 (26.2856, 67) -> (26.2856, 63)
  line L741 (30.2856, 67) -> (26.2856, 67)
  line L742 (30.2856, 59) -> (26.2856, 59)
  line L743 (26.2856, 59) -> (26.2856, 55)
  line L744 (30.2856, 55) -> (30.2856, 59)
  line L745 (26.2856, 55) -> (30.2856, 55)
  line L746 (30.2856, 51) -> (26.2856, 51)
  line L747 (26.2856, 51) -> (26.2856, 47)
  line L748 (26.2856, 47) -> (30.2856, 47)
  line L749 (30.2856, 47) -> (30.2856, 51)
  line L750 (30.2856, 43) -> (26.2856, 43)
  line L751 (26.2856, 43) -> (26.2856, 39)
  line L752 (30.2856, 39) -> (30.2856, 43)
  line L753 (26.2856, 39) -> (30.2856, 39)
  line L754 (30.2856, 35) -> (26.2856, 35)
  line L755 (30.2856, 31) -> (30.2856, 35)
  line L756 (26.2856, 31) -> (30.2856, 31)
  line L757 (26.2856, 35) -> (26.2856, 31)
  line L758 (30.2856, 27) -> (26.2856, 27)
  line L759 (26.2856, 27) -> (26.2856, 23)
  line L760 (30.2856, 23) -> (30.2856, 27)
  line L761 (26.2856, 23) -> (30.2856, 23)
  line L762 (30.2856, 19) -> (26.2856, 19)
  line L763 (26.2856, 19) -> (26.2856, 15)
  line L764 (26.2856, 15) -> (30.2856, 15)
  line L765 (30.2856, 15) -> (30.2856, 19)
  line L766 (30.2856, 11) -> (26.2856, 11)
  line L767 (26.2856, 11) -> (26.2856, 7)
  line L768 (26.2856, 7) -> (30.2856, 7)
  line L769 (30.2856, 7) -> (30.2856, 11)
  line L770 (22.2856, 127) -> (22.2856, 131)
  line L771 (22.2856, 131) -> (18.2856, 131)
  line L772 (18.2856, 131) -> (18.2856, 127)
  line L773 (18.2856, 123) -> (18.2856, 119)
  line L774 (18.2856, 119) -> (22.2856, 119)
  line L775 (22.2856, 119) -> (22.2856, 123)
  line L776 (22.2856, 115) -> (18.2856, 115)
  line L777 (22.2856, 111) -> (22.2856, 115)
  line L778 (18.2856, 115) -> (18.2856, 111)
  line L779 (18.2856, 111) -> (22.2856, 111)
  line L780 (22.2856, 107) -> (18.2856, 107)
  line L781 (18.2856, 103) -> (22.2856, 103)
  line L782 (18.2856, 107) -> (18.2856, 103)
  line L783 (22.2856, 103) -> (22.2856, 107)
  line L784 (18.2856, 127) -> (22.2856, 127)
  line L785 (22.2856, 123) -> (18.2856, 123)
  line L786 (22.2856, 99) -> (18.2856, 99)
  line L787 (18.2856, 99) -> (18.2856, 95)
  line L788 (22.2856, 95) -> (22.2856, 99)
  line L789 (22.2856, 91) -> (18.2856, 91)
  line L790 (18.2856, 87) -> (22.2856, 87)
  line L791 (22.2856, 87) -> (22.2856, 91)
  line L792 (18.2856, 91) -> (18.2856, 87)
  line L793 (18.2856, 95) -> (22.2856, 95)
  line L794 (22.2856, 83) -> (18.2856, 83)
  line L795 (18.2856, 83) -> (18.2856, 79)
  line L796 (22.2856, 79) -> (22.2856, 83)
  line L797 (18.2856, 79) -> (22.2856, 79)
  line L798 (22.2856, 75) -> (18.2856, 75)
  line L799 (18.2856, 75) -> (18.2856, 71)
  line L800 (22.2856, 71) -> (22.2856, 75)
  line L801 (18.2856, 71) -> (22.2856, 71)
  line L802 (18.2856, 63) -> (22.2856, 63)
  line L803 (22.2856, 63) -> (22.2856, 67)
  line L804 (18.2856, 67) -> (18.2856, 63)
  line L805 (22.2856, 67) -> (18.2856, 67)
  line L806 (22.2856, 59) -> (18.2856, 59)
  line L807 (18.2856, 59) -> (18.2856, 55)
  line L808 (22.2856, 55) -> (22.2856, 59)
  line L809 (18.2856, 55) -> (22.2856, 55)
  line L810 (22.2856, 51) -> (18.2856, 51)
  line L811 (18.2856, 51) -> (18.2856, 47)
  line L812 (18.2856, 47) -> (22.2856, 47)
  line L813 (22.2856, 47) -> (22.2856, 51)
  line L814 (22.2856, 43) -> (18.2856, 43)
  line L815 (18.2856, 43) -> (18.2856, 39)
  line L816 (22.2856, 39) -> (22.2856, 43)
  line L817 (18.2856, 39) -> (22.2856, 39)
  line L818 (22.2856, 35) -> (18.2856, 35)
  line L819 (22.2856, 31) -> (22.2856, 35)
  line L820 (18.2856, 31) -> (22.2856, 31)
  line L821 (18.2856, 35) -> (18.2856, 31)
  line L822 (22.2856, 27) -> (18.2856, 27)
  line L823 (18.2856, 27) -> (18.2856, 23)
  line L824 (22.2856, 23) -> (22.2856, 27)
  line L825 (18.2856, 23) -> (22.2856, 23)
  line L826 (22.2856, 19) -> (18.2856, 19)
  line L827 (18.2856, 19) -> (18.2856, 15)
  line L828 (18.2856, 15) -> (22.2856, 15)
  line L829 (22.2856, 15) -> (22.2856, 19)
  line L830 (22.2856, 11) -> (18.2856, 11)
  line L831 (18.2856, 11) -> (18.2856, 7)
  line L832 (18.2856, 7) -> (22.2856, 7)
  line L833 (22.2856, 7) -> (22.2856, 11)
  line L834 (14.2856, 127) -> (14.2856, 131)
  line L835 (14.2856, 131) -> (10.2856, 131)
  line L836 (10.2856, 131) -> (10.2856, 127)
  line L837 (10.2856, 123) -> (10.2856, 119)
  line L838 (10.2856, 119) -> (14.2856, 119)
  line L839 (14.2856, 119) -> (14.2856, 123)
  line L840 (14.2856, 115) -> (10.2856, 115)
  line L841 (14.2856, 111) -> (14.2856, 115)
  line L842 (10.2856, 115) -> (10.2856, 111)
  line L843 (10.2856, 111) -> (14.2856, 111)
  line L844 (14.2856, 107) -> (10.2856, 107)
  line L845 (10.2856, 103) -> (14.2856, 103)
  line L846 (10.2856, 107) -> (10.2856, 103)
  line L847 (14.2856, 103) -> (14.2856, 107)
  line L848 (10.2856, 127) -> (14.2856, 127)
  line L849 (14.2856, 123) -> (10.2856, 123)
  line L850 (14.2856, 99) -> (10.2856, 99)
  line L851 (10.2856, 99) -> (10.2856, 95)
  line L852 (14.2856, 95) -> (14.2856, 99)
  line L853 (14.2856, 91) -> (10.2856, 91)
  line L854 (10.2856, 87) -> (14.2856, 87)
  line L855 (14.2856, 87) -> (14.2856, 91)
  line L856 (10.2856, 91) -> (10.2856, 87)
  line L857 (10.2856, 95) -> (14.2856, 95)
  line L858 (14.2856, 83) -> (10.2856, 83)
  line L859 (10.2856, 83) -> (10.2856, 79)
  line L860 (14.2856, 79) -> (14.2856, 83)
  line L861 (10.2856, 79) -> (14.2856, 79)
  line L862 (14.2856, 75) -> (10.2856, 75)
  line L863 (10.2856, 75) -> (10.2856, 71)
  line L864 (14.2856, 71) -> (14.2856, 75)
  line L865 (10.2856, 71) -> (14.2856, 71)
  line L866 (10.2856, 63) -> (14.2856, 63)
  line L867 (14.2856, 63) -> (14.2856, 67)
  line L868 (10.2856, 67) -> (10.2856, 63)
  line L869 (14.2856, 67) -> (10.2856, 67)
  line L870 (14.2856, 59) -> (10.2856, 59)
  line L871 (10.2856, 59) -> (10.2856, 55)
  line L872 (14.2856, 55) -> (14.2856, 59)
  line L873 (10.2856, 55) -> (14.2856, 55)
  line L874 (14.2856, 51) -> (10.2856, 51)
  line L875 (10.2856, 51) -> (10.2856, 47)
  line L876 (10.2856, 47) -> (14.2856, 47)
  line L877 (14.2856, 47) -> (14.2856, 51)
  line L878 (14.2856, 43) -> (10.2856, 43)
  line L879 (10.2856, 43) -> (10.2856, 39)
  line L880 (14.2856, 39) -> (14.2856, 43)
  line L881 (10.2856, 39) -> (14.2856, 39)
  line L882 (14.2856, 35) -> (10.2856, 35)
  line L883 (14.2856, 31) -> (14.2856, 35)
  line L884 (10.2856, 31) -> (14.2856, 31)
  line L885 (10.2856, 35) -> (10.2856, 31)
  line L886 (14.2856, 27) -> (10.2856, 27)
  line L887 (10.2856, 27) -> (10.2856, 23)
  line L888 (14.2856, 23) -> (14.2856, 27)
  line L889 (10.2856, 23) -> (14.2856, 23)
  line L890 (14.2856, 19) -> (10.2856, 19)
  line L891 (10.2856, 19) -> (10.2856, 15)
  line L892 (10.2856, 15) -> (14.2856, 15)
  line L893 (14.2856, 15) -> (14.2856, 19)
  line L894 (14.2856, 11) -> (10.2856, 11)
  line L895 (10.2856, 11) -> (10.2856, 7)
  line L896 (10.2856, 7) -> (14.2856, 7)
  line L897 (14.2856, 7) -> (14.2856, 11)
  point P0 (54.1438, 139)
  dimension "d73" = 4
  dimension "d74" = 4
  dimension "d75" = 6
  dimension "d76" = 8
  dimension "d79" = 8
  dimension "d86" = 8
  constraints: 1792 end point, 2 horizontal, 2 parallel, 1 perpendicular, 1 vertical, 1784 other
  measures "d73" distance of L1.end L2.end
  measures "d74" distance of L0.end L1.end
  measures "d75" distance between parallel lines of L4 L3
  measures "d76" distance between parallel lines of L5 L0
  measures "d79" distance of L0.start L6.start
  measures "d86" distance of L0.start L66.end
extrude "Extrusión6" cut sketch "Boceto7" against normal up to surface (5 mm away)
equation "\"d62\" = d66"
equation "\"d68\" = d65"
equation "\"d74\" = d73"
